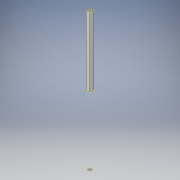
# Autodesk Inventor part: corner
Saved by Autodesk Inventor 2018 (Build 220112000, 112)
## iProperties
Created: 2018-11-24
Part Number: corner
Material: Generic
Document SubType Name: Modeling
Designer: Gage
Density: 1 g/cm^3
Appearance: Default
Author: Gage
Autodesk Inventor part; units mm, degrees
ref_plane "YZ Plane" through (0, 0, 0) normal (1, 0, 0) x (0, 1, 0)
ref_plane "XZ Plane" through (0, 0, 0) normal (0, 1, 0) x (-1, 0, 0)
ref_plane "XY Plane" through (0, 0, 0) normal (0, 0, 1) x (1, 0, 0)
sketch "Sketch1" plane through (0, 0, 0) normal (0, 0, 1) x (1, 0, 0)
  line L0 (-0.6985, 30.861) -> (0.6985, 30.861)
  line L1 (0.6985, 30.861) -> (0.6985, -30.861)
  line L2 (0.6985, -30.861) -> (-0.6985, -30.861)
  line L3 (-0.6985, -30.861) -> (-0.6985, 30.861)
  line L4 (-0.6985, 30.861) -> (0.6985, -30.861) construction
  line L5 (0.6985, 30.861) -> (-0.6985, -30.861) construction
  point P0 (0, 0)
  dimension "d0" = 1.397
  dimension "d1" = 61.722
  constraints: 12 end point, 2 midpoint, 2 parallel, 1 horizontal, 1 perpendicular
  measures "d0" distance of L1.end L2.end
  measures "d1" distance of L0.end L1.end
extrude "Extrusion1" add sketch "Sketch1" along normal blind 1.397
sketch "Sketch3" plane through (0.6985, -30.861, 0) normal (1, 0, 0) x (0, 0, -1)
  line L0 (0, 61.722) -> (0, 0) projected
  line L1 (0, 61.722) -> (-1.397, 61.722) projected
  line L2 (-1.397, 0) -> (-1.397, 61.722) projected
  line L3 (0, 0) -> (-1.397, 0) projected
  line L4 (-1.397, 0) -> (-1.905, 0)
  line L5 (-1.397, 0) -> (-1.397, 1.27)
  line L6 (-1.397, 53.34) -> (-1.397, 0) projected
  line L7 (-1.651, 1.27) -> (-1.397, 1.27)
  line L8 (-1.651, 1.27) -> (-1.905, 0)
  point P0 (0, 30.861)
  dimension "d8" = 0.508
  dimension "d9" = 1.27
  dimension "d10" = 0.254
  constraints: 8 end point, 2 horizontal, 1 collinear
  measures "d8" distance of L2.start L4.end
  measures "d9" distance of L2.start L5.end
  measures "d10" distance of L7.start L5.end
ref_plane "Work Plane2" through (-0.6985, -30.226, 0) normal (0, -1, 0) x (1, 0, 0)
sketch "Sketch7" plane through (-0.6985, -30.226, 0) normal (0, -1, 0) x (1, 0, 0)
  line L0 (1.3985, 1.651) -> (-0.254, 1.651)
  line L1 (-0.254, 1.651) -> (-0.254, 0)
  line L2 (0, 0) -> (0, 1.397) projected
  line L3 (0, 1.397) -> (1.397, 1.397) projected
  point P0 (0.6985, 0)
  dimension "d20" = 0.254
  dimension "d21" = 0.254
  constraints: 4 end point, 1 horizontal, 1 perpendicular
  measures "d20" distance between parallel lines of L1 L2
  measures "d21" distance between parallel lines of L3 L0
sweep "Sweep2" add profiles "Sketch3" path "Sketch7" path curves L0 L1 contours L4 L8 L7 L2
ref_plane "Work Plane4" through (-0.6985, 20.574, 0) normal (0, -1, 0) x (1, 0, 0)
ref_plane "Work Plane3" through (-0.6985, -4.826, 0) normal (0, -1, 0) x (1, 0, 0)
split "Split1" plane through (-0.6985, -4.826, 0) removes the side toward (0, -1, 0)
split "Split2" plane through (-0.6985, 20.574, 0) removes the side toward (0, 1, 0)
body "Solid1"
